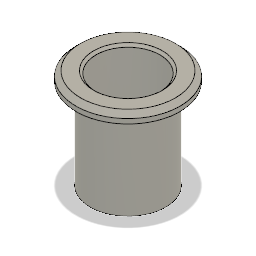
Router Bit Holder (Autodesk Fusion 360 design; units mm, degrees)
Autodesk Fusion 360 part; units mm, degrees
sketch "Sketch1" plane through (0, 0, 0) normal (0, 0, 1) x (1, 0, 0)
  line L0 (0, 0) -> (-8, 0)
  line L1 (-8, 0) -> (-8, 19)
  line L2 (-8, 19) -> (0, 19)
  line L3 (0, 19) -> (0, 0)
  line L4 (0, 19) -> (-6.75, 19)
  line L5 (-6.75, 19) -> (-6.75, 7)
  line L6 (-6.75, 7) -> (0, 7)
  line L7 (0, 7) -> (0, 19)
  line L8 (0, 7) -> (-3.5, 7)
  line L9 (-3.5, 7) -> (-3.5, 1)
  line L10 (-3.5, 1) -> (0, 1)
  line L11 (0, 1) -> (0, 7)
  line L12 (0, 19) -> (-11, 19)
  line L13 (-11, 19) -> (-11, 21)
  line L14 (-11, 21) -> (0, 21)
  line L15 (0, 21) -> (0, 19)
  line L16 (-6.75, 19) -> (-6.75, 21)
  line L17 (0, 1) -> (-1, 1)
  line L18 (-1, 1) -> (-1, 0)
  line L19 (-1, 0) -> (0, 0)
  line L20 (0, 0) -> (0, 1)
  dimension "d1" = 19
  dimension "d2" = 8
  dimension "d7" = 12
  dimension "d8" = 6.75
  dimension "d9" = 6
  dimension "d10" = 3.5
  dimension "d11" = 11
  dimension "d12" = 2
  measures "d1" distance of L0.start
  measures "d2" distance of L0.start
  measures "d9" distance of L0.start
  measures "d12" distance of L0.start
revolve "Revolve1" add sketch "Sketch1" angle 360 about axis through (0, 19, 0) along (0, -1, 0) contours L0 L1 L2 L5 L6 L9 L10 L12 L18 | L2 L12 L13 L14 L16
chamfer "Chamfer1" distance 1 angle 45 1 edges at (-10.2556, 21, 3.9778)
chamfer "Chamfer2" distance 0.5 angle 45 1 edges at (-6.2932, 21, 2.4409)
chamfer "Chamfer3" distance 2 angle 15 1 edges at (-6.2932, 7, 2.4409) measured on face at (-5.6285, 7, 0.5092)
chamfer "Chamfer4" distance 1 angle 30 1 edges at (-3.2631, 1, 1.2657) measured on face at (-2.6499, 1, 0.2236)
equation "d2 = Width / 2"
equation "Height = 19 mm"
equation "Width = 16 mm"
equation "LargeShank = 13.5 mm"
equation "SmallShank = 7 mm"
equation "d8 = LargeShank / 2"
equation "d10 = SmallShank / 2"
